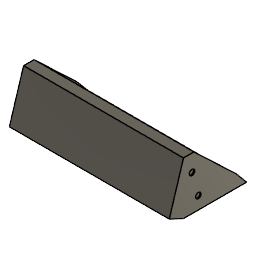
Bucket v2 (Autodesk Fusion 360 design; units mm, degrees)
Autodesk Fusion 360 part; units mm, degrees
note: some values were not read from the file. Set by a fixed rule: which sketch regions a step uses.
sketch "Sketch1" plane through (0, 0, 0) normal (1, 0, 0) x (0, 1, 0)
  line L0 (0, 0) -> (60, 0)
  line L1 (60, 0) -> (49.9725, 11.9503)
  line L2 (49.9725, 11.9503) -> (9.9318, 49.9475)
  line L3 (49.9725, 11.9503) -> (105.1725, 11.9503) construction
  line L4 (9.9318, 49.9475) -> (-0.0682, 49.9475)
  line L5 (0, 0) -> (-13.5946, 6.3393)
  line L6 (0, 0) -> (15, 0) construction
  line L7 (-13.5946, 6.3393) -> (-0.0682, 49.9475)
  dimension "d15" = 60
  dimension "d16" = 15.6
  dimension "d18" = 136.5
  dimension "d19" = 55.2
  dimension "d24" = 155
  dimension "d25" = 15
  constraint coincident L0.start L5.start
  constraint horizontal L0
  constraint horizontal L3
  constraint horizontal L4
  constraint horizontal L6
  measures "d15" distance of L0.start L0.end
  measures "d16" distance of L0.end L1.end
  measures "d18" angle of L2 L3
  measures "d19" distance of L1.end L2.end
  measures "d24" angle of L5 L6
  measures "d25" distance of L0.start L5.end
extrude "Extrude1" add sketch "Sketch1" along normal mid plane 152
shell "Shell1" thickness 1 removed faces 2 at (25.3333, 23.2787, 37.2817) at (25.3333, 56.6575, 3.9834)
sketch "Sketch3" plane through (0, -14.1952, 4.4031) normal (0, -0.955108, 0.296257) x (1, 0, 0)
  line L0 (-76, 2.0272) -> (76, 2.0272)
  line L1 (76, 2.0272) -> (76, 47.685)
  line L2 (76, 47.685) -> (-76, 47.685)
  line L3 (-76, 47.685) -> (-76, 2.0272)
  line L4 (0, 2.0272) -> (0, 47.685)
  line L5 (-69, 24.0272) -> (-69, 33.0272)
  line L6 (-69, 24.0272) -> (-69, 15.0272)
  line L7 (-69, 33.0272) -> (-51, 33.0272)
  line L8 (-51, 33.0272) -> (-51, 15.0272)
  line L9 (-51, 15.0272) -> (-69, 15.0272)
  line L10 (69, 33.0272) -> (51, 33.0272)
  line L11 (51, 33.0272) -> (51, 15.0272)
  line L12 (51, 15.0272) -> (69, 15.0272)
  line L13 (69, 24.0272) -> (69, 15.0272)
  line L14 (69, 24.0272) -> (69, 33.0272)
  constraint midpoint L0 L4.start
  constraint midpoint L2 L4.end
  constraint perpendicular L5 L7
  constraint symmetric L4 L5.start L13.start
  constraint symmetric L4 L5.end L10.start
  constraint symmetric L4 L6.end L12.end
  constraint symmetric L4 L7.end L10.end
  constraint symmetric L4 L8.end L11.end
extrude "Extrude3" add sketch "Sketch3" along normal blind 28 contours L5 L6 L7 L8 L9 | L10 L11 L12 L13 L14
sketch "Sketch4" plane through (0, -40.9382, 12.6983) normal (0, -0.955108, 0.296257) x (1, 0, 0)
  line L0 (-69, 33.0272) -> (-69, 15.0272)
  line L1 (-69, 15.0272) -> (-51, 15.0272)
  line L2 (-51, 15.0272) -> (-51, 33.0272)
  line L3 (-51, 33.0272) -> (-69, 33.0272)
  line L4 (-54.8, 30.2) -> (-65.2, 30.2)
  line L5 (-65.2, 30.2) -> (-65.2, 17.8)
  line L6 (-65.2, 17.8) -> (-54.8, 17.8)
  line L7 (-54.8, 17.8) -> (-54.8, 30.2)
  line L8 (-54.8, 30.2) -> (-65.2, 17.8) construction
  line L9 (-65.2, 30.2) -> (-54.8, 17.8) construction
  line L10 (54.8, 30.2) -> (65.2, 17.8) construction
  line L11 (65.2, 30.2) -> (54.8, 17.8) construction
  line L12 (65.2, 30.2) -> (65.2, 17.8)
  line L13 (65.2, 17.8) -> (54.8, 17.8)
  line L14 (54.8, 17.8) -> (54.8, 30.2)
  line L15 (54.8, 30.2) -> (65.2, 30.2)
  point P0 (-60, 24)
  point P1 (60, 24)
  dimension "d50" = 10.4
  dimension "d51" = 12.4
  constraint horizontal L4
  constraint perpendicular L4 L5
  constraint parallel L4 L6
  constraint parallel L5 L7
  constraint coincident L8 P0
  constraint coincident L9 P0
  measures "d50" distance of L5.end L6.end
  measures "d51" distance of L4.end L5.end
extrude "Extrude4" cut sketch "Sketch4" against normal blind 28.2 contours L4 L5 L6 L7 | L12 L13 L14 L15
delete_face "DeleteFace1" 10 faces at (69, -16.8801, 27.2514) (57, -18.6576, 21.5207) (52.2667, -33.2104, 37.6121) (63, -22.2393, 41.4778) (51, -25.7944, 30.0165) (-69, -16.8801, 27.2514) (-57, -18.6576, 21.5207) (-52.2667, -33.2104, 37.6121) (-63, -13.325, 38.7127) (-51, -25.7944, 30.0165)
extrude "Extrude5" add 2 faces at (61.7333, -7.5063, 25.2925) (-58.2667, -7.5063, 25.2925) along direction (0, -0.955108, 0.296257) blind 0.2
sketch "Sketch5" plane through (76, 0, 0) normal (1, 0, 0) x (0, 1, 0)
  line L0 (0, 0) -> (60, 0)
  line L1 (60, 0) -> (49.9725, 11.9503)
  line L2 (49.9725, 11.9503) -> (9.9318, 49.9475)
  line L3 (9.9318, 49.9475) -> (-0.0682, 49.9475)
  line L4 (-0.0682, 49.9475) -> (-13.5946, 6.3393)
  line L5 (-13.5946, 6.3393) -> (0, 0)
  circle A0 centre (14, 12) radius 2.6
  circle A1 centre (8, 34) radius 2.6
  dimension "d58" = 5.2
  dimension "d60" = 5.2
  measures "d58" diameter of A0
  measures "d60" diameter of A1
extrude "Extrude6" cut sketch "Sketch5" against normal through all contours A0 | A1
extrude "Extrude2" [suppressed]
equation "bucket_width = 152 mm"
equation "bucket_depth = 60 mm"
equation "bucket_back_height = 50 mm"
equation "wall = 4.5 mm"
equation "side_wall = 5.5 mm"
equation "lip = 7 mm"
equation "pivot_ear_thickness = 6 mm"
equation "pivot_hole = 5 mm"
equation "top_flange = 8 mm"
